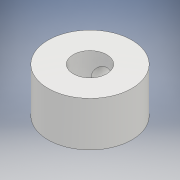
# Autodesk Inventor part: ジュラコンセットカラー061508
Saved by Autodesk Inventor 2017 (Build 210142000, 142)
## iProperties
Part Number: ジュラコンセットカラー061508
Material: アセタール樹脂、白
Document SubType Name: Modeling
Designer: 雪村
Density: 1.425 g/cm^3
Appearance: 滑らか - 白
Author: 雪村
Autodesk Inventor part; units mm, degrees
ref_plane "YZ Plane" through (0, 0, 0) normal (1, 0, 0) x (0, 1, 0)
ref_plane "XZ Plane" through (0, 0, 0) normal (0, 1, 0) x (-1, 0, 0)
ref_plane "XY Plane" through (0, 0, 0) normal (0, 0, 1) x (1, 0, 0)
sketch "スケッチ1" plane through (0, 0, 0) normal (0, 0, 1) x (1, 0, 0)
  circle A0 centre (0, 0) radius 3
  circle A1 centre (0, 0) radius 7.5
  dimension "d0" = 6
  dimension "d1" = 15
  constraints: 2 centre point, 2 coincident
  measures "d0" diameter of A0
  measures "d1" diameter of A1
extrude "押し出し1" add sketch "スケッチ1" along normal blind 8
sketch "スケッチ2" plane through (0, 0, 0) normal (0, 1, 0) x (-1, 0, 0)
  line L0 (7.5, 8) -> (-7.5, 8) projected
  line L1 (-7.5, 0) -> (7.5, 0) projected
  line L2 (-3, 0) -> (-3, 8) projected
  line L3 (3, 0) -> (3, 8) projected
  circle A0 centre (0, 4) radius 2
  point P0 (0, 0)
  dimension "d4" = 4
  dimension "d5" = 4
  dimension "d6" = 3
  constraints: 1 centre point
  measures "d4" diameter of A0
  measures "d5" distance from line of L0 A0.centre
  measures "d6" distance from line of L2 A0.centre
extrude "押し出し2" cut sketch "スケッチ2" along normal through all contours A0
